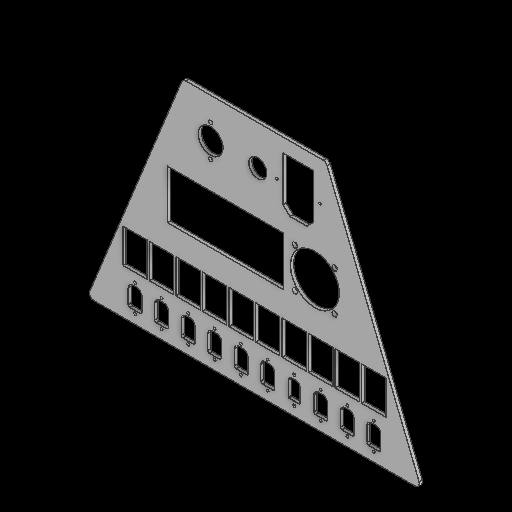
# Autodesk Inventor part: BreakerMount
Saved by Autodesk Inventor 2025.2 (Build 292293000, 293)
## iProperties
Created: 2025-11-18
Part Number: BreakerMount
Material: Generic
Document SubType Name: Sheet Metal
Designer: valer
Density: 1 g/cm^3
Sheet Metal Rule: Default
Appearance: Default
Author: valer
Autodesk Inventor part; units mm, degrees
ref_plane "YZ Plane" through (0, 0, 0) normal (1, 0, 0) x (0, 1, 0)
ref_plane "XZ Plane" through (0, 0, 0) normal (0, 1, 0) x (-1, 0, 0)
ref_plane "XY Plane" through (0, 0, 0) normal (0, 0, 1) x (1, 0, 0)
sketch "Base" plane through (0, 0, 0) normal (0, 0, 1) x (1, 0, 0)
  line L0 (0, 0) -> (70.3402, 0)
  line L1 (70.3402, 0) -> (183.2019, -220)
  line L2 (183.2019, -220) -> (0, -220)
  line L3 (0, -220) -> (0, 0) construction
  line L4 (0, 0) -> (-70.3402, 0)
  line L5 (-70.3402, 0) -> (-183.2019, -220)
  line L6 (-183.2019, -220) -> (0, -220)
  line L7 (-63.3831, 22.3248) -> (-182.4251, -209.7225) construction
  dimension "d1" = 220
  dimension "d3" = 4
  measures "d1" distance between parallel lines of L6 L4
  measures "d3" distance between parallel lines of L7 L5
extrude "Plate1" add sketch "Base" along normal blind 3
fillet "FilletsFeature" radius 6 4 edges at (-70.3402, 0, 1.5) (70.3402, 0, 1.5) (183.2019, -220, 1.5) (-183.2019, -220, 1.5)
sketch "MatchProduction" plane through (0, 0, 3) normal (0, 0, 1) x (1, 0, 0)
  line L0 (0, -264.1502) -> (0, 44.901) construction
  line L1 (-66.6748, 0) -> (66.6748, 0) projected
  line L2 (66.6748, 0) -> (155.5606, -220)
  line L3 (173.3804, -220) -> (-173.3804, -220) projected
  arc A0 (72.0133, -3.2613) -> (66.6748, 0) centre (66.6748, -6) ccw projected
  line L4 (72.0133, -3.2613) -> (178.7189, -211.2613) projected
  arc A1 (173.3804, -220) -> (178.7189, -211.2613) centre (173.3804, -214) ccw projected
  arc A2 (-178.7189, -211.2613) -> (-173.3804, -220) centre (-173.3804, -214) ccw projected
  line L5 (-178.7189, -211.2613) -> (-72.0133, -3.2613) projected
  arc A3 (-66.6748, 0) -> (-72.0133, -3.2613) centre (-66.6748, -6) ccw projected
  line L6 (-66.6748, 0) -> (-155.5606, -220)
  point P0 (0, 0)
  point P1 (-155.5606, -220)
  dimension "d13" = 68
  constraints: 4 end point, 1 point on line, 1 symmetric about line
  measures "d13" angle of L3 L2
extrude "MatchProductionFeature" cut sketch "MatchProduction" against normal blind 3 contours L6 L3 A2 L5 A3 | A0 L4 A1 L3 L2
fillet "OutsideFilletsFeature" radius 4 4 edges at (-155.5606, -220, 1.5) (155.5606, -220, 1.5) (66.6748, 0, 1.5) (-66.6748, 0, 1.5)
sketch "MeterMountHoles" plane through (0, 0, 0) normal (0, 0, -1) x (-1, 0, 0)
  circle A0 centre (-37.8, -81.5) radius 2.5 projected
  circle A1 centre (-37.8, -118.5) radius 2.5 projected
  circle A2 centre (-74.8, -118.5) radius 2.5 projected
  circle A3 centre (-74.8, -81.5) radius 2.5 projected
  circle A4 centre (-56.3, -100) radius 22.5 construction
  line L0 (80.8, -122.5) -> (80.8, -77.5) construction
  line L1 (80.8, -77.5) -> (26.8, -77.5) construction
  line L2 (26.8, -122.5) -> (80.8, -122.5) construction
  line L3 (26.8, -77.5) -> (26.8, -122.5) construction
  line L4 (0.05, -122.575) -> (26.8, -122.575) construction
  line L5 (26.8, -77.425) -> (0.05, -77.425) construction
  line L6 (-26.8, -122.575) -> (-0.05, -122.575) construction
  line L7 (-0.05, -77.425) -> (-26.8, -77.425) construction
  line L8 (-26.8, -122.575) -> (-26.8, -77.425) construction
  line L9 (26.8, -122.575) -> (80.8, -122.575) construction
  line L10 (80.8, -122.575) -> (80.8, -122.5)
  line L11 (80.8, -77.5) -> (80.8, -77.425)
  line L12 (80.8, -77.425) -> (26.8, -77.425) construction
  line L13 (80.8, -122.575) -> (-26.8, -122.575)
  line L14 (-26.8, -122.575) -> (-26.8, -77.425)
  line L15 (-26.8, -77.425) -> (80.8, -77.425)
  circle A5 centre (-56.3, -100) radius 23
  point P0 (0, 0)
  dimension "d62" = 0.5
  constraints: 16 end point, 3 perpendicular, 2 collinear, 2 horizontal, 1 centre point, 1 parallel, 1 vertical
  measures "d62" radial gap between concentric circles of A4 A5
extrude "MeterMountHolesFeature" cut sketch "MeterMountHoles" against normal blind 3 contours A0 | A1 | A2 | A3
sketch "ExpandHole" plane through (0, 0, 0) normal (0, 0, -1) x (-1, 0, 0)
  circle A0 centre (-74.8, -81.5) radius 2.5 construction
  circle A1 centre (-37.8, -81.5) radius 2.5 construction
  circle A2 centre (-74.8, -118.5) radius 2.5 construction
  circle A3 centre (-37.8, -118.5) radius 2.5 construction
  arc A4 (67.6855, -2.5016) -> (63.9768, 0) centre (63.9768, -4) ccw projected
  line L0 (-63.9768, 0) -> (63.9768, 0) projected
  arc A5 (-63.9768, 0) -> (-67.6855, -2.5016) centre (-63.9768, -4) ccw projected
  line L1 (-67.6855, -2.5016) -> (-153.339, -214.5016) projected
  arc A6 (-153.339, -214.5016) -> (-149.6303, -220) centre (-149.6303, -216) ccw projected
  line L2 (149.6303, -220) -> (-149.6303, -220) projected
  arc A7 (149.6303, -220) -> (153.339, -214.5016) centre (149.6303, -216) ccw projected
  line L3 (153.339, -214.5016) -> (67.6855, -2.5016) projected
  circle A8 centre (-56.3, -100) radius 22.75
  circle A9 centre (-56.3, -100) radius 22.5 construction
  point P0 (0, 0)
  dimension "d63" = 0.25
  constraints: 1 centre point, 1 coincident
  measures "d63" radial gap between concentric circles of A8 A9
extrude "ExpandHoleFeature" cut sketch "ExpandHole" against normal blind 3 contours A8
sketch "PowerHub" plane through (0, 0, 3) normal (0, 0, 1) x (1, 0, 0)
  arc A0 (-40.8, -25.675) -> (-40.8, -47.925) centre (-40.8, -36.8) ccw construction
  arc A1 (-40.8, -47.925) -> (-40.8, -25.675) centre (-40.8, -36.8) ccw construction
  circle A2 centre (3.2, -36.8) radius 8 construction
  line L0 (33.2, -60.295) -> (27.2, -54.295) construction
  line L1 (48.632, -60.295) -> (33.2, -60.295) construction
  line L2 (54.632, -54.295) -> (48.632, -60.295) construction
  line L3 (54.632, -13.305) -> (54.632, -54.295) construction
  line L4 (27.2, -13.305) -> (54.632, -13.305) construction
  line L5 (27.2, -54.295) -> (27.2, -13.305) construction
  line L6 (104.5044, -150.7) -> (117.7956, -150.7) construction
  line L7 (117.7956, -150.7) -> (117.7956, -173.7) construction
  line L8 (117.7956, -173.7) -> (104.5044, -173.7) construction
  line L9 (104.5044, -173.7) -> (104.5044, -150.7) construction
  line L10 (121.945, -146.85) -> (100.355, -146.85) construction
  line L11 (100.355, -146.85) -> (100.355, -177.55) construction
  line L12 (100.355, -177.55) -> (121.945, -177.55) construction
  line L13 (121.945, -177.55) -> (121.945, -146.85) construction
  line L14 (79.8044, -150.7) -> (93.0956, -150.7) construction
  line L15 (93.0956, -150.7) -> (93.0956, -173.7) construction
  line L16 (93.0956, -173.7) -> (79.8044, -173.7) construction
  line L17 (79.8044, -173.7) -> (79.8044, -150.7) construction
  line L18 (97.245, -146.85) -> (75.655, -146.85) construction
  line L19 (75.655, -146.85) -> (75.655, -177.55) construction
  line L20 (75.655, -177.55) -> (97.245, -177.55) construction
  line L21 (97.245, -177.55) -> (97.245, -146.85) construction
  line L22 (55.1044, -150.7) -> (68.3956, -150.7) construction
  line L23 (68.3956, -150.7) -> (68.3956, -173.7) construction
  line L24 (68.3956, -173.7) -> (55.1044, -173.7) construction
  line L25 (55.1044, -173.7) -> (55.1044, -150.7) construction
  line L26 (72.545, -146.85) -> (50.955, -146.85) construction
  line L27 (50.955, -146.85) -> (50.955, -177.55) construction
  line L28 (50.955, -177.55) -> (72.545, -177.55) construction
  line L29 (72.545, -177.55) -> (72.545, -146.85) construction
  line L30 (30.4044, -150.7) -> (43.6956, -150.7) construction
  line L31 (43.6956, -150.7) -> (43.6956, -173.7) construction
  line L32 (43.6956, -173.7) -> (30.4044, -173.7) construction
  line L33 (30.4044, -173.7) -> (30.4044, -150.7) construction
  line L34 (47.845, -146.85) -> (26.255, -146.85) construction
  line L35 (26.255, -146.85) -> (26.255, -177.55) construction
  line L36 (26.255, -177.55) -> (47.845, -177.55) construction
  line L37 (47.845, -177.55) -> (47.845, -146.85) construction
  line L38 (5.7044, -150.7) -> (18.9956, -150.7) construction
  line L39 (18.9956, -150.7) -> (18.9956, -173.7) construction
  line L40 (18.9956, -173.7) -> (5.7044, -173.7) construction
  line L41 (5.7044, -173.7) -> (5.7044, -150.7) construction
  line L42 (23.145, -146.85) -> (1.555, -146.85) construction
  line L43 (1.555, -146.85) -> (1.555, -177.55) construction
  line L44 (1.555, -177.55) -> (23.145, -177.55) construction
  line L45 (23.145, -177.55) -> (23.145, -146.85) construction
  line L46 (-18.9956, -150.7) -> (-5.7044, -150.7) construction
  line L47 (-5.7044, -150.7) -> (-5.7044, -173.7) construction
  line L48 (-5.7044, -173.7) -> (-18.9956, -173.7) construction
  line L49 (-18.9956, -173.7) -> (-18.9956, -150.7) construction
  line L50 (-1.555, -146.85) -> (-23.145, -146.85) construction
  line L51 (-23.145, -146.85) -> (-23.145, -177.55) construction
  line L52 (-23.145, -177.55) -> (-1.555, -177.55) construction
  line L53 (-1.555, -177.55) -> (-1.555, -146.85) construction
  line L54 (-43.6956, -150.7) -> (-30.4044, -150.7) construction
  line L55 (-30.4044, -150.7) -> (-30.4044, -173.7) construction
  line L56 (-30.4044, -173.7) -> (-43.6956, -173.7) construction
  line L57 (-43.6956, -173.7) -> (-43.6956, -150.7) construction
  line L58 (-26.255, -146.85) -> (-47.845, -146.85) construction
  line L59 (-47.845, -146.85) -> (-47.845, -177.55) construction
  line L60 (-47.845, -177.55) -> (-26.255, -177.55) construction
  line L61 (-26.255, -177.55) -> (-26.255, -146.85) construction
  line L62 (-68.3956, -150.7) -> (-55.1044, -150.7) construction
  line L63 (-55.1044, -150.7) -> (-55.1044, -173.7) construction
  line L64 (-55.1044, -173.7) -> (-68.3956, -173.7) construction
  line L65 (-68.3956, -173.7) -> (-68.3956, -150.7) construction
  line L66 (-50.955, -146.85) -> (-72.545, -146.85) construction
  line L67 (-72.545, -146.85) -> (-72.545, -177.55) construction
  line L68 (-72.545, -177.55) -> (-50.955, -177.55) construction
  line L69 (-50.955, -177.55) -> (-50.955, -146.85) construction
  line L70 (-93.0956, -150.7) -> (-79.8044, -150.7) construction
  line L71 (-79.8044, -150.7) -> (-79.8044, -173.7) construction
  line L72 (-79.8044, -173.7) -> (-93.0956, -173.7) construction
  line L73 (-93.0956, -173.7) -> (-93.0956, -150.7) construction
  line L74 (-75.655, -146.85) -> (-97.245, -146.85) construction
  line L75 (-97.245, -146.85) -> (-97.245, -177.55) construction
  line L76 (-97.245, -177.55) -> (-75.655, -177.55) construction
  line L77 (-75.655, -177.55) -> (-75.655, -146.85) construction
  line L78 (-117.7956, -150.7) -> (-104.5044, -150.7) construction
  line L79 (-104.5044, -150.7) -> (-104.5044, -173.7) construction
  line L80 (-104.5044, -173.7) -> (-117.7956, -173.7) construction
  line L81 (-117.7956, -173.7) -> (-117.7956, -150.7) construction
  line L82 (-100.355, -146.85) -> (-121.945, -146.85) construction
  line L83 (-121.945, -146.85) -> (-121.945, -177.55) construction
  line L84 (-121.945, -177.55) -> (-100.355, -177.55) construction
  line L85 (-100.355, -177.55) -> (-100.355, -146.85) construction
  circle A3 centre (-111.15, -195.5) radius 2.5 construction
  circle A4 centre (-111.15, -202.5) radius 2.5 construction
  arc A5 (-105.25, -193.55) -> (-109.05, -189.75) centre (-109.05, -193.55) ccw construction
  line L86 (-109.05, -189.75) -> (-113.25, -189.75) construction
  arc A6 (-113.25, -189.75) -> (-117.05, -193.55) centre (-113.25, -193.55) ccw construction
  line L87 (-117.05, -193.55) -> (-117.05, -207.25) construction
  arc A7 (-117.05, -207.25) -> (-116.05, -208.25) centre (-116.05, -207.25) ccw construction
  line L88 (-116.05, -208.25) -> (-106.25, -208.25) construction
  arc A8 (-106.25, -208.25) -> (-105.25, -207.25) centre (-106.25, -207.25) ccw construction
  line L89 (-105.25, -207.25) -> (-105.25, -193.55) construction
  circle A9 centre (-86.45, -195.5) radius 2.5 construction
  circle A10 centre (-86.45, -202.5) radius 2.5 construction
  arc A11 (-80.55, -193.55) -> (-84.35, -189.75) centre (-84.35, -193.55) ccw construction
  line L90 (-84.35, -189.75) -> (-88.55, -189.75) construction
  arc A12 (-88.55, -189.75) -> (-92.35, -193.55) centre (-88.55, -193.55) ccw construction
  line L91 (-92.35, -193.55) -> (-92.35, -207.25) construction
  arc A13 (-92.35, -207.25) -> (-91.35, -208.25) centre (-91.35, -207.25) ccw construction
  line L92 (-91.35, -208.25) -> (-81.55, -208.25) construction
  arc A14 (-81.55, -208.25) -> (-80.55, -207.25) centre (-81.55, -207.25) ccw construction
  line L93 (-80.55, -207.25) -> (-80.55, -193.55) construction
  circle A15 centre (-61.75, -195.5) radius 2.5 construction
  circle A16 centre (-61.75, -202.5) radius 2.5 construction
  arc A17 (-55.85, -193.55) -> (-59.65, -189.75) centre (-59.65, -193.55) ccw construction
  line L94 (-59.65, -189.75) -> (-63.85, -189.75) construction
  arc A18 (-63.85, -189.75) -> (-67.65, -193.55) centre (-63.85, -193.55) ccw construction
  line L95 (-67.65, -193.55) -> (-67.65, -207.25) construction
  arc A19 (-67.65, -207.25) -> (-66.65, -208.25) centre (-66.65, -207.25) ccw construction
  line L96 (-66.65, -208.25) -> (-56.85, -208.25) construction
  arc A20 (-56.85, -208.25) -> (-55.85, -207.25) centre (-56.85, -207.25) ccw construction
  line L97 (-55.85, -207.25) -> (-55.85, -193.55) construction
  circle A21 centre (-37.05, -195.5) radius 2.5 construction
  circle A22 centre (-37.05, -202.5) radius 2.5 construction
  arc A23 (-31.15, -193.55) -> (-34.95, -189.75) centre (-34.95, -193.55) ccw construction
  line L98 (-34.95, -189.75) -> (-39.15, -189.75) construction
  arc A24 (-39.15, -189.75) -> (-42.95, -193.55) centre (-39.15, -193.55) ccw construction
  line L99 (-42.95, -193.55) -> (-42.95, -207.25) construction
  arc A25 (-42.95, -207.25) -> (-41.95, -208.25) centre (-41.95, -207.25) ccw construction
  line L100 (-41.95, -208.25) -> (-32.15, -208.25) construction
  arc A26 (-32.15, -208.25) -> (-31.15, -207.25) centre (-32.15, -207.25) ccw construction
  line L101 (-31.15, -207.25) -> (-31.15, -193.55) construction
  circle A27 centre (-12.35, -195.5) radius 2.5 construction
  circle A28 centre (-12.35, -202.5) radius 2.5 construction
  arc A29 (-6.45, -193.55) -> (-10.25, -189.75) centre (-10.25, -193.55) ccw construction
  line L102 (-10.25, -189.75) -> (-14.45, -189.75) construction
  arc A30 (-14.45, -189.75) -> (-18.25, -193.55) centre (-14.45, -193.55) ccw construction
  line L103 (-18.25, -193.55) -> (-18.25, -207.25) construction
  arc A31 (-18.25, -207.25) -> (-17.25, -208.25) centre (-17.25, -207.25) ccw construction
  line L104 (-17.25, -208.25) -> (-7.45, -208.25) construction
  arc A32 (-7.45, -208.25) -> (-6.45, -207.25) centre (-7.45, -207.25) ccw construction
  line L105 (-6.45, -207.25) -> (-6.45, -193.55) construction
  circle A33 centre (12.35, -195.5) radius 2.5 construction
  circle A34 centre (12.35, -202.5) radius 2.5 construction
  arc A35 (18.25, -193.55) -> (14.45, -189.75) centre (14.45, -193.55) ccw construction
  line L106 (14.45, -189.75) -> (10.25, -189.75) construction
  arc A36 (10.25, -189.75) -> (6.45, -193.55) centre (10.25, -193.55) ccw construction
  line L107 (6.45, -193.55) -> (6.45, -207.25) construction
  arc A37 (6.45, -207.25) -> (7.45, -208.25) centre (7.45, -207.25) ccw construction
  line L108 (7.45, -208.25) -> (17.25, -208.25) construction
  arc A38 (17.25, -208.25) -> (18.25, -207.25) centre (17.25, -207.25) ccw construction
  line L109 (18.25, -207.25) -> (18.25, -193.55) construction
  circle A39 centre (37.05, -195.5) radius 2.5 construction
  circle A40 centre (37.05, -202.5) radius 2.5 construction
  arc A41 (42.95, -193.55) -> (39.15, -189.75) centre (39.15, -193.55) ccw construction
  line L110 (39.15, -189.75) -> (34.95, -189.75) construction
  arc A42 (34.95, -189.75) -> (31.15, -193.55) centre (34.95, -193.55) ccw construction
  line L111 (31.15, -193.55) -> (31.15, -207.25) construction
  arc A43 (31.15, -207.25) -> (32.15, -208.25) centre (32.15, -207.25) ccw construction
  line L112 (32.15, -208.25) -> (41.95, -208.25) construction
  arc A44 (41.95, -208.25) -> (42.95, -207.25) centre (41.95, -207.25) ccw construction
  line L113 (42.95, -207.25) -> (42.95, -193.55) construction
  circle A45 centre (61.75, -195.5) radius 2.5 construction
  circle A46 centre (61.75, -202.5) radius 2.5 construction
  arc A47 (67.65, -193.55) -> (63.85, -189.75) centre (63.85, -193.55) ccw construction
  line L114 (63.85, -189.75) -> (59.65, -189.75) construction
  arc A48 (59.65, -189.75) -> (55.85, -193.55) centre (59.65, -193.55) ccw construction
  line L115 (55.85, -193.55) -> (55.85, -207.25) construction
  arc A49 (55.85, -207.25) -> (56.85, -208.25) centre (56.85, -207.25) ccw construction
  line L116 (56.85, -208.25) -> (66.65, -208.25) construction
  arc A50 (66.65, -208.25) -> (67.65, -207.25) centre (66.65, -207.25) ccw construction
  line L117 (67.65, -207.25) -> (67.65, -193.55) construction
  circle A51 centre (86.45, -195.5) radius 2.5 construction
  circle A52 centre (86.45, -202.5) radius 2.5 construction
  arc A53 (92.35, -193.55) -> (88.55, -189.75) centre (88.55, -193.55) ccw construction
  line L118 (88.55, -189.75) -> (84.35, -189.75) construction
  arc A54 (84.35, -189.75) -> (80.55, -193.55) centre (84.35, -193.55) ccw construction
  line L119 (80.55, -193.55) -> (80.55, -207.25) construction
  arc A55 (80.55, -207.25) -> (81.55, -208.25) centre (81.55, -207.25) ccw construction
  line L120 (81.55, -208.25) -> (91.35, -208.25) construction
  arc A56 (91.35, -208.25) -> (92.35, -207.25) centre (91.35, -207.25) ccw construction
  line L121 (92.35, -207.25) -> (92.35, -193.55) construction
  circle A57 centre (111.15, -195.5) radius 2.5 construction
  circle A58 centre (111.15, -202.5) radius 2.5 construction
  arc A59 (117.05, -193.55) -> (113.25, -189.75) centre (113.25, -193.55) ccw construction
  line L122 (113.25, -189.75) -> (109.05, -189.75) construction
  arc A60 (109.05, -189.75) -> (105.25, -193.55) centre (109.05, -193.55) ccw construction
  line L123 (105.25, -193.55) -> (105.25, -207.25) construction
  arc A61 (105.25, -207.25) -> (106.25, -208.25) centre (106.25, -207.25) ccw construction
  line L124 (106.25, -208.25) -> (116.05, -208.25) construction
  arc A62 (116.05, -208.25) -> (117.05, -207.25) centre (116.05, -207.25) ccw construction
  line L125 (117.05, -207.25) -> (117.05, -193.55) construction
  line L126 (55.132, -54.5021) -> (48.8391, -60.795)
  line L127 (48.8391, -60.795) -> (32.9929, -60.795)
  line L128 (32.9929, -60.795) -> (26.7, -54.5021)
  line L129 (26.7, -54.5021) -> (26.7, -12.805)
  line L130 (26.7, -12.805) -> (55.132, -12.805)
  line L131 (55.132, -12.805) -> (55.132, -54.5021)
  circle A63 centre (3.2, -36.8) radius 8.5
  arc A64 (-40.8, -25.175) -> (-40.8, -48.425) centre (-40.8, -36.8) ccw
  arc A65 (-40.8, -48.425) -> (-40.8, -25.175) centre (-40.8, -36.8) ccw
  line L132 (99.855, -178.05) -> (99.855, -146.35)
  line L133 (99.855, -146.35) -> (122.445, -146.35)
  line L134 (122.445, -146.35) -> (122.445, -178.05)
  line L135 (122.445, -178.05) -> (99.855, -178.05)
  line L136 (75.155, -146.35) -> (97.745, -146.35)
  line L137 (97.745, -146.35) -> (97.745, -178.05)
  line L138 (97.745, -178.05) -> (75.155, -178.05)
  line L139 (75.155, -178.05) -> (75.155, -146.35)
  line L140 (50.455, -146.35) -> (73.045, -146.35)
  line L141 (73.045, -146.35) -> (73.045, -178.05)
  line L142 (73.045, -178.05) -> (50.455, -178.05)
  line L143 (50.455, -178.05) -> (50.455, -146.35)
  line L144 (25.755, -146.35) -> (48.345, -146.35)
  line L145 (48.345, -146.35) -> (48.345, -178.05)
  line L146 (48.345, -178.05) -> (25.755, -178.05)
  line L147 (25.755, -178.05) -> (25.755, -146.35)
  line L148 (1.055, -146.35) -> (23.645, -146.35)
  line L149 (23.645, -146.35) -> (23.645, -178.05)
  line L150 (23.645, -178.05) -> (1.055, -178.05)
  line L151 (1.055, -178.05) -> (1.055, -146.35)
  line L152 (-23.645, -146.35) -> (-1.055, -146.35)
  line L153 (-1.055, -146.35) -> (-1.055, -178.05)
  line L154 (-1.055, -178.05) -> (-23.645, -178.05)
  line L155 (-23.645, -178.05) -> (-23.645, -146.35)
  line L156 (-48.345, -146.35) -> (-25.755, -146.35)
  line L157 (-25.755, -146.35) -> (-25.755, -178.05)
  line L158 (-25.755, -178.05) -> (-48.345, -178.05)
  line L159 (-48.345, -178.05) -> (-48.345, -146.35)
  line L160 (-73.045, -146.35) -> (-50.455, -146.35)
  line L161 (-50.455, -146.35) -> (-50.455, -178.05)
  line L162 (-50.455, -178.05) -> (-73.045, -178.05)
  line L163 (-73.045, -178.05) -> (-73.045, -146.35)
  line L164 (-97.745, -146.35) -> (-75.155, -146.35)
  line L165 (-75.155, -146.35) -> (-75.155, -178.05)
  line L166 (-75.155, -178.05) -> (-97.745, -178.05)
  line L167 (-97.745, -178.05) -> (-97.745, -146.35)
  line L168 (-122.445, -146.35) -> (-99.855, -146.35)
  line L169 (-99.855, -146.35) -> (-99.855, -178.05)
  line L170 (-99.855, -178.05) -> (-122.445, -178.05)
  line L171 (-122.445, -178.05) -> (-122.445, -146.35)
  arc A66 (-113.25, -189.25) -> (-117.55, -193.55) centre (-113.25, -193.55) ccw
  line L172 (-113.25, -189.25) -> (-109.05, -189.25)
  arc A67 (-104.75, -193.55) -> (-109.05, -189.25) centre (-109.05, -193.55) ccw
  line L173 (-104.75, -193.55) -> (-104.75, -207.25)
  arc A68 (-106.25, -208.75) -> (-104.75, -207.25) centre (-106.25, -207.25) ccw
  line L174 (-106.25, -208.75) -> (-116.05, -208.75)
  arc A69 (-117.55, -207.25) -> (-116.05, -208.75) centre (-116.05, -207.25) ccw
  line L175 (-117.55, -207.25) -> (-117.55, -193.55)
  arc A70 (-88.55, -189.25) -> (-92.85, -193.55) centre (-88.55, -193.55) ccw
  line L176 (-88.55, -189.25) -> (-84.35, -189.25)
  arc A71 (-80.05, -193.55) -> (-84.35, -189.25) centre (-84.35, -193.55) ccw
  line L177 (-80.05, -193.55) -> (-80.05, -207.25)
  arc A72 (-81.55, -208.75) -> (-80.05, -207.25) centre (-81.55, -207.25) ccw
  line L178 (-81.55, -208.75) -> (-91.35, -208.75)
  arc A73 (-92.85, -207.25) -> (-91.35, -208.75) centre (-91.35, -207.25) ccw
  line L179 (-92.85, -207.25) -> (-92.85, -193.55)
  arc A74 (-63.85, -189.25) -> (-68.15, -193.55) centre (-63.85, -193.55) ccw
  line L180 (-63.85, -189.25) -> (-59.65, -189.25)
  arc A75 (-55.35, -193.55) -> (-59.65, -189.25) centre (-59.65, -193.55) ccw
  line L181 (-55.35, -193.55) -> (-55.35, -207.25)
  arc A76 (-56.85, -208.75) -> (-55.35, -207.25) centre (-56.85, -207.25) ccw
  line L182 (-56.85, -208.75) -> (-66.65, -208.75)
  arc A77 (-68.15, -207.25) -> (-66.65, -208.75) centre (-66.65, -207.25) ccw
  line L183 (-68.15, -207.25) -> (-68.15, -193.55)
  arc A78 (-39.15, -189.25) -> (-43.45, -193.55) centre (-39.15, -193.55) ccw
  line L184 (-39.15, -189.25) -> (-34.95, -189.25)
  arc A79 (-30.65, -193.55) -> (-34.95, -189.25) centre (-34.95, -193.55) ccw
  line L185 (-30.65, -193.55) -> (-30.65, -207.25)
  arc A80 (-32.15, -208.75) -> (-30.65, -207.25) centre (-32.15, -207.25) ccw
  line L186 (-32.15, -208.75) -> (-41.95, -208.75)
  arc A81 (-43.45, -207.25) -> (-41.95, -208.75) centre (-41.95, -207.25) ccw
  line L187 (-43.45, -207.25) -> (-43.45, -193.55)
  arc A82 (-14.45, -189.25) -> (-18.75, -193.55) centre (-14.45, -193.55) ccw
  line L188 (-14.45, -189.25) -> (-10.25, -189.25)
  arc A83 (-5.95, -193.55) -> (-10.25, -189.25) centre (-10.25, -193.55) ccw
  line L189 (-5.95, -193.55) -> (-5.95, -207.25)
  arc A84 (-7.45, -208.75) -> (-5.95, -207.25) centre (-7.45, -207.25) ccw
  line L190 (-7.45, -208.75) -> (-17.25, -208.75)
  arc A85 (-18.75, -207.25) -> (-17.25, -208.75) centre (-17.25, -207.25) ccw
  line L191 (-18.75, -207.25) -> (-18.75, -193.55)
  arc A86 (10.25, -189.25) -> (5.95, -193.55) centre (10.25, -193.55) ccw
  line L192 (10.25, -189.25) -> (14.45, -189.25)
  arc A87 (18.75, -193.55) -> (14.45, -189.25) centre (14.45, -193.55) ccw
  line L193 (18.75, -193.55) -> (18.75, -207.25)
  arc A88 (17.25, -208.75) -> (18.75, -207.25) centre (17.25, -207.25) ccw
  line L194 (17.25, -208.75) -> (7.45, -208.75)
  arc A89 (5.95, -207.25) -> (7.45, -208.75) centre (7.45, -207.25) ccw
  line L195 (5.95, -207.25) -> (5.95, -193.55)
  line L196 (34.95, -190.25) -> (39.15, -190.25)
  arc A90 (42.45, -193.55) -> (39.15, -190.25) centre (39.15, -193.55) ccw
  line L197 (42.45, -193.55) -> (42.45, -207.25)
  arc A91 (41.95, -207.75) -> (42.45, -207.25) centre (41.95, -207.25) ccw
  line L198 (41.95, -207.75) -> (32.15, -207.75)
  arc A92 (31.65, -207.25) -> (32.15, -207.75) centre (32.15, -207.25) ccw
  line L199 (31.65, -207.25) -> (31.65, -193.55)
  arc A93 (34.95, -190.25) -> (31.65, -193.55) centre (34.95, -193.55) ccw
  line L200 (55.35, -207.25) -> (55.35, -193.55)
  arc A94 (59.65, -189.25) -> (55.35, -193.55) centre (59.65, -193.55) ccw
  line L201 (59.65, -189.25) -> (63.85, -189.25)
  arc A95 (68.15, -193.55) -> (63.85, -189.25) centre (63.85, -193.55) ccw
  line L202 (68.15, -193.55) -> (68.15, -207.25)
  arc A96 (66.65, -208.75) -> (68.15, -207.25) centre (66.65, -207.25) ccw
  line L203 (66.65, -208.75) -> (56.85, -208.75)
  arc A97 (55.35, -207.25) -> (56.85, -208.75) centre (56.85, -207.25) ccw
  arc A98 (84.35, -189.25) -> (80.05, -193.55) centre (84.35, -193.55) ccw
  line L204 (84.35, -189.25) -> (88.55, -189.25)
  arc A99 (92.85, -193.55) -> (88.55, -189.25) centre (88.55, -193.55) ccw
  line L205 (92.85, -193.55) -> (92.85, -207.25)
  arc A100 (91.35, -208.75) -> (92.85, -207.25) centre (91.35, -207.25) ccw
  line L206 (91.35, -208.75) -> (81.55, -208.75)
  arc A101 (80.05, -207.25) -> (81.55, -208.75) centre (81.55, -207.25) ccw
  line L207 (80.05, -207.25) -> (80.05, -193.55)
  line L208 (109.05, -189.25) -> (113.25, -189.25)
  arc A102 (117.55, -193.55) -> (113.25, -189.25) centre (113.25, -193.55) ccw
  line L209 (117.55, -193.55) -> (117.55, -207.25)
  arc A103 (116.05, -208.75) -> (117.55, -207.25) centre (116.05, -207.25) ccw
  line L210 (116.05, -208.75) -> (106.25, -208.75)
  arc A104 (104.75, -207.25) -> (106.25, -208.75) centre (106.25, -207.25) ccw
  line L211 (104.75, -207.25) -> (104.75, -193.55)
  arc A105 (109.05, -189.25) -> (104.75, -193.55) centre (109.05, -193.55) ccw
  point P0 (0, 0)
  dimension "d37" = 0.5
  dimension "d38" = 0.5
  dimension "d39" = 0.5
  dimension "d40" = 0.5
  dimension "d41" = 0.5
  dimension "d42" = 0.5
  dimension "d43" = 0.5
  dimension "d44" = 0.5
  dimension "d45" = 0.5
  dimension "d46" = 0.5
  dimension "d47" = 0.5
  dimension "d48" = 0.5
  dimension "d49" = 0.5
  dimension "d50" = 0.5
  dimension "d51" = 0.5
  dimension "d52" = 0.5
  dimension "d53" = 0.5
  dimension "d54" = 0.5
  dimension "d55" = 0.5
  dimension "d56" = 0.5
  dimension "d57" = 0.5
  dimension "d58" = 0.5
  dimension "d59" = 0.5
  constraints: 172 end point, 84 point on circle, 43 centre point, 106 other
  measures "d37" distance between parallel lines of L3 L131
  measures "d38" radial gap between concentric circles of A2 A63
  measures "d39" radial gap between concentric circles of A1 A65
  measures "d40" distance between parallel lines of L11 L132
  measures "d41" distance between parallel lines of L18 L136
  measures "d42" distance between parallel lines of L26 L140
  measures "d43" distance between parallel lines of L34 L144
  measures "d44" distance between parallel lines of L42 L148
  measures "d45" distance between parallel lines of L50 L152
  measures "d46" distance between parallel lines of L58 L156
  measures "d47" distance between parallel lines of L66 L160
  measures "d48" distance between parallel lines of L74 L164
  measures "d49" distance between parallel lines of L82 L168
  measures "d50" radial gap between concentric circles of A6 A66
  measures "d51" radial gap between concentric circles of A12 A70
  measures "d52" radial gap between concentric circles of A18 A74
  measures "d53" radial gap between concentric circles of A24 A78
  measures "d54" radial gap between concentric circles of A30 A82
  measures "d55" radial gap between concentric circles of A36 A86
  measures "d56" distance between parallel lines of L110 L196
  measures "d57" distance between parallel lines of L115 L200
  measures "d58" radial gap between concentric circles of A54 A98
  measures "d59" distance between parallel lines of L122 L208
extrude "PowerHubFeature" cut sketch "PowerHub" against normal blind 3
sketch "PaneMeters2" plane through (0, 0, 0) normal (0, 0, -1) x (-1, 0, 0)
  line L0 (78.3, -120) -> (29.3, -120) construction
  line L1 (29.3, -120) -> (29.3, -80) construction
  line L2 (29.3, -80) -> (78.3, -80) construction
  line L3 (78.3, -80) -> (78.3, -120) construction
  line L4 (80.8, -77.5) -> (26.8, -77.5) construction
  line L5 (26.8, -77.5) -> (26.8, -122.5) construction
  line L6 (26.8, -122.5) -> (80.8, -122.5) construction
  line L7 (80.8, -122.5) -> (80.8, -77.5) construction
  line L8 (26.8, -77.425) -> (0.05, -77.425) construction
  line L9 (-0.05, -77.425) -> (-26.8, -77.425) construction
  line L10 (-26.8, -79.425) -> (-26.8, -102.575) construction
  line L11 (-26.8, -122.575) -> (-0.05, -122.575) construction
  line L12 (0.05, -122.575) -> (26.8, -122.575) construction
  line L13 (81.05, -122.825) -> (-27.05, -122.825)
  line L14 (-27.05, -122.825) -> (-27.05, -77.25)
  line L15 (-27.05, -77.25) -> (81.05, -77.25)
  line L16 (81.05, -77.25) -> (81.05, -122.825)
  point P0 (0, 0)
  dimension "d64" = 0.25
  dimension "d65" = 0.25
  dimension "d66" = 0.25
  dimension "d67" = 0.25
  constraints: 8 end point, 2 parallel, 1 horizontal, 1 perpendicular
  measures "d64" distance between parallel lines of L15 L4
  measures "d65" distance between parallel lines of L16 L7
  measures "d66" distance between parallel lines of L14 L10
  measures "d67" distance between parallel lines of L13 L11
extrude "PanelMeters2Feature" cut sketch "PaneMeters2" against normal blind 3
sketch "MountHoles" plane through (0, 0, 0) normal (0, 0, -1) x (-1, 0, 0)
  circle A0 centre (-20.916, -36.8) radius 1.75 construction
  circle A1 centre (-60.916, -36.8) radius 1.75 construction
  circle A2 centre (-20.916, -36.8) radius 1.3
  circle A3 centre (-60.916, -36.8) radius 1.3
  circle A4 centre (111.15, -211.5) radius 1.55 construction
  circle A5 centre (111.15, -186.5) radius 1.55 construction
  circle A6 centre (86.45, -211.5) radius 1.55 construction
  circle A7 centre (86.45, -186.5) radius 1.55 construction
  circle A8 centre (61.75, -211.5) radius 1.55 construction
  circle A9 centre (61.75, -186.5) radius 1.55 construction
  circle A10 centre (37.05, -211.5) radius 1.55 construction
  circle A11 centre (37.05, -186.5) radius 1.55 construction
  circle A12 centre (12.35, -211.5) radius 1.55 construction
  circle A13 centre (12.35, -186.5) radius 1.55 construction
  circle A14 centre (-12.35, -211.5) radius 1.55 construction
  circle A15 centre (-12.35, -186.5) radius 1.55 construction
  circle A16 centre (-37.05, -211.5) radius 1.55 construction
  circle A17 centre (-37.05, -186.5) radius 1.55 construction
  circle A18 centre (-61.75, -211.5) radius 1.55 construction
  circle A19 centre (-61.75, -186.5) radius 1.55 construction
  circle A20 centre (-86.45, -211.5) radius 1.55 construction
  circle A21 centre (-86.45, -186.5) radius 1.55 construction
  circle A22 centre (-111.15, -211.5) radius 1.55 construction
  circle A23 centre (-111.15, -186.5) radius 1.55 construction
  circle A24 centre (111.15, -211.5) radius 1.3
  circle A25 centre (111.15, -186.5) radius 1.3
  circle A26 centre (86.45, -211.5) radius 1.3
  circle A27 centre (86.45, -186.5) radius 1.3
  circle A28 centre (61.75, -211.5) radius 1.3
  circle A29 centre (61.75, -186.5) radius 1.3
  circle A30 centre (37.05, -186.5) radius 1.3
  circle A31 centre (37.05, -211.5) radius 1.3
  circle A32 centre (12.35, -211.5) radius 1.3
  circle A33 centre (12.35, -186.5) radius 1.3
  circle A34 centre (-12.35, -211.5) radius 1.3
  circle A35 centre (-12.35, -186.5) radius 1.3
  circle A36 centre (-37.05, -211.5) radius 1.3
  circle A37 centre (-37.05, -186.5) radius 1.3
  circle A38 centre (-61.75, -211.5) radius 1.3
  circle A39 centre (-61.75, -186.5) radius 1.3
  circle A40 centre (-86.45, -211.5) radius 1.3
  circle A41 centre (-86.45, -186.5) radius 1.3
  circle A42 centre (-111.15, -211.5) radius 1.3
  circle A43 centre (-111.15, -186.5) radius 1.3
  circle A44 centre (40.8, -51.8) radius 2 construction
  circle A45 centre (40.8, -21.8) radius 2 construction
  circle A46 centre (40.8, -51.8) radius 1.8
  circle A47 centre (40.8, -21.8) radius 1.8
  point P0 (0, 0)
  dimension "d70" = 2.6
  dimension "d71" = 2.6
  dimension "d72" = 2.6
  dimension "d73" = 2.6
  dimension "d74" = 2.6
  dimension "d75" = 2.6
  dimension "d78" = 4
  dimension "d79" = 3.6
  dimension "d80" = 3.6
  constraints: 24 centre point, 24 coincident, 16 equal radius
  measures "d70" diameter of A2
  measures "d71" diameter of A3
  measures "d72" diameter of A24
  measures "d73" diameter of A25
  measures "d74" diameter of A26
  measures "d75" diameter of A27
  measures "d78" diameter of A44
  measures "d79" diameter of A46
  measures "d80" diameter of A47
extrude "MountHolesFeature" cut sketch "MountHoles" against normal blind 3
equation "\"d14\" = Thickness"
equation "\"d17\" = Thickness"
equation "\"d33\" = Thickness"
equation "\"d60\" = Thickness"
equation "\"d68\" = Thickness"
equation "\"d76\" = Thickness"
equation "\"d0\" = Thickness"
equation "\"BendRadius\" = Thickness"
equation "\"BendReliefWidth\" = Thickness"
equation "\"BendReliefDepth\" = 0.5 * Thickness"
equation "\"CornerReliefSize\" = 4 * Thickness"
equation "\"MinimumRemnant\" = 2 * Thickness"
equation "\"TransitionRadius\" = BendRadius"
equation "\"JacobiRadiusSize\" = BendRadius"
equation "\"GapSize\" = Thickness"
equation "\"Thickness\" = 3"
body "Solid1"
